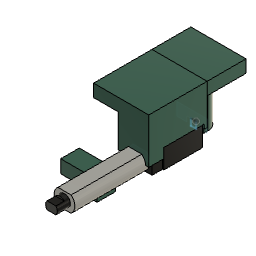
Actuator Casing (Autodesk Fusion 360 design; units mm, degrees)
Autodesk Fusion 360 part; units mm, degrees
note: some values were not read from the file. Chosen so that the rebuilt part matches the saved one: which bodies a step acts on; which pieces of a blend or face edit are solid. Set by a fixed rule: which sketch regions a step uses.
sketch "Sketch4" plane through (0, 0, 0) normal (0, 1, 0) x (1, 0, 0)
  line L0 (-5.3517, 0.0536) -> (-5.3517, 0) construction
  line L1 (-5.1362, -6.1335) -> (5.1362, -6.1335)
  line L2 (5.1029, 6.1612) -> (-5.1029, 6.1612)
  arc A0 (5.1362, -6.1335) -> (5.1029, 6.1612) centre (0, 0) ccw
  arc A1 (-5.1029, 6.1612) -> (-5.1362, -6.1335) centre (0, 0) ccw
  line L3 (-3.4975, -0.0044) -> (-3.4975, -3.0044) construction
  line L4 (-3.3853, -2.9647) -> (3.3222, -2.9647)
  line L5 (3.3222, 3.0353) -> (-3.3853, 3.0353)
  line L6 (-3.3853, 3.0353) -> (-3.3853, 2.9647)
  line L7 (-9.0073, 0.0216) -> (-9.0073, -7.4784) construction
  line L8 (0, 0) -> (-9.5, 0) construction
  line L9 (-9.5, 0) -> (-9.5, -7.4784) construction
  line L10 (-9.5, -7.4784) -> (9.5, -7.4784)
  line L11 (9.5, -7.4784) -> (9.5, 7.5216)
  line L12 (9.5, 7.5216) -> (-9.5, 7.5216)
  line L13 (-9.5, 7.5216) -> (-9.5, -7.4784)
  line L14 (-9.5, 7.5216) -> (-9.5, -7.4784)
  arc A2 (3.3853, -2.9647) -> (3.3222, 3.0353) centre (0, 0) ccw
  arc A3 (-3.3222, 3.0353) -> (-3.3853, -2.9647) centre (0, 0) ccw
  line L15 (3.3222, -2.9647) -> (3.3853, -2.9647)
  circle A4 centre (0, 0) radius 4.5
  line L16 (9.5, 7.5216) -> (10.5, 7.5216)
  line L17 (10.5, 7.5216) -> (10.5, -7.4784)
  line L18 (10.5, -7.4784) -> (9.5, -7.4784)
  line L19 (9.5, -7.4784) -> (9.5, 7.5216)
  dimension "d21" = 16
  dimension "d23" = 9
  dimension "d24" = 3
  dimension "d25" = 6
  dimension "d26" = 7.5
  dimension "d27" = 9.5
  dimension "d28" = 19
  dimension "d29" = 15
  dimension "d31" = 15
  dimension "d34" = 9
  dimension "d85" = 1
  dimension "d86" = 15
  constraint coincident A0.centre A1.centre
  constraint vertical L0
  constraint horizontal L1
  constraint horizontal L2
  constraint concentric A0 A1
  constraint vertical L3
  constraint horizontal L4
  constraint horizontal L5
  constraint vertical L6
  constraint vertical L7
  constraint perpendicular L7 L8
  constraint perpendicular L8 L9
  constraint horizontal L10
  constraint vertical L11
  constraint horizontal L12
  constraint vertical L13
  constraint vertical L14
  constraint coincident L4 A2.start
  constraint coincident L6.end A2
  constraint coincident L5 A3.start
  constraint concentric A2 A3
  constraint coincident L8 L0.end
  constraint concentric A1 A4
  constraint horizontal L16
  constraint vertical L17
  constraint horizontal L18
  constraint vertical L19
  measures "d21" diameter of A0
  measures "d23" diameter of A2
  measures "d24" distance of L3.start L3.end
  measures "d25" distance of L4.start L5.end
  measures "d26" distance of L7.start L7.end
  measures "d27" distance of A0.centre L8.end
  measures "d28" distance of L9.end L10.end
  measures "d29" distance of L9.end L12.end
  measures "d31" distance of L9.end L12.end
  measures "d34" diameter of A4
  measures "d85" distance of L11.end L16.end
  measures "d86" distance of L11.end L10.end
extrude "Extrude9" add sketch "Sketch4" against normal blind 68 contours L4 L5 A2 A3 L15 A4 makes body 1
extrude "Extrude10" add sketch "Sketch4" against normal blind 61.5 contours L4 L15 A4 | L5 A4 bodies 1
extrude "Extrude11" add sketch "Sketch4" against normal blind 58 contours L1 L2 A0 A1 bodies 1
extrude "Extrude12" add sketch "Sketch4" along normal blind 38 contours L10 L11 L12 L13 L14 L19 bodies 1
extrude "Extrude13" add sketch "Sketch4" along normal blind 30 from surface at 8 contours L1 L2 A0 A1 | L10 L11 L12 L13 L14 L19 | L11 L16 L17 L18 L19 bodies 1
sketch "Sketch5" plane through (0, 0, 0) normal (0, 0, 1) x (1, 0, 0)
  circle A0 centre (0, 43) radius 2.15
  line L0 (-5, 38) -> (-5, 43)
  line L1 (5, 38) -> (5, 43)
  arc A1 (5, 43) -> (-5, 43) centre (0, 43) ccw
  line L2 (-5, 38) -> (5, 38)
  dimension "d53" = 10
  dimension "d54" = 4.3
  constraint concentric A0 A1
  constraint tangent L0 A1
  constraint tangent L1 A1
  constraint horizontal L2
  measures "d53" diameter of A1
  measures "d54" diameter of A0
extrude "Extrude14" add sketch "Sketch5" along normal blind 4 and the other way blind 4 bodies 1
sketch "Sketch6" plane through (0, 38, 0) normal (0, 1, 0) x (-1, 0, 0)
  line L0 (9.5, 7.4784) -> (-10.5, 7.4784)
  line L1 (-10.5, -7.5216) -> (9.5, -7.5216)
  line L2 (9.5, 7.4784) -> (-10.5, 7.4784)
  line L3 (-10.5, 7.4784) -> (-10.5, -7.5216)
  line L4 (-10.5, -7.5216) -> (9.5, -7.5216)
  line L5 (9.5, -7.5216) -> (9.5, 7.4784)
  arc A0 (2.0616, 4) -> (-2.0616, 4) centre (0, 0) ccw
  line L6 (-5, 4) -> (-2.0616, 4)
  line L7 (2.0616, 4) -> (5, 4)
  line L8 (5, 4) -> (5, -4)
  line L9 (5, -4) -> (2.0616, -4)
  arc A1 (-2.0616, -4) -> (2.0616, -4) centre (0, 0) ccw
  line L10 (-2.0616, -4) -> (-5, -4)
  line L11 (-5, -4) -> (-5, 4)
  line L12 (-10.5, 7.4784) -> (-10.5, -7.5216)
  line L13 (9.5, -7.5216) -> (9.5, 7.4784)
  constraint horizontal L2
  constraint vertical L3
  constraint horizontal L4
  constraint vertical L5
  constraint coincident L1.start L3.end
  constraint coincident L0.start L2.start
sketch "Sketch7" plane through (0, 0, 2.9647) normal (0, 0, 1) x (-1, 0, 0)
  line L0 (-3.3853, 61.5) -> (3.3853, 61.5)
  line L1 (3.3853, 61.5) -> (3.3853, 68)
  line L2 (3.3853, 68) -> (-3.3853, 68)
  line L3 (-3.3853, 68) -> (-3.3853, 61.5)
copy_body "Body->Comp1" bodies 1 removing the originals makes body 2 in component "actuator"
sketch "Sketch5 (2)" plane through (0, 0, 0) normal (0, 0, 1) x (1, 0, 0) in component "casing 1"
  line L0 (13, 0) -> (-12, 0)
  line L1 (13, 38) -> (-12, 38)
  line L2 (-10, -58) -> (10.3853, -58)
  constraint horizontal L0
  constraint horizontal L1
  constraint horizontal L2
split "Split2" by plane through (0, 0, 0) normal (0, 1, 0) bodies 2 makes body 3 at (-3.1667, 15.3333, 7.4784) in component "actuator"
sketch "Sketch1" plane through (0, 0, 6.1335) normal (0, 0, 1) x (-1, 0, 0) in component "actuator"
  line L0 (-5.1362, 0) -> (5.1362, 0)
  line L1 (5.1362, 0) -> (5.1362, 58)
  line L2 (5.1362, 58) -> (-5.1362, 58)
  line L3 (-5.1362, 58) -> (-5.1362, 0)
  line L4 (-10.7245, 58) -> (12, 58)
  constraint horizontal L4
split "Split3" by curves path "Sketch1" along L4 bodies 2 makes body 4 at (-5.4286, -19.3333, 5.8763) in component "actuator"
sketch "Sketch2" plane through (0, 0, 7.4784) normal (0, 0, 1) x (-1, 0, 0) in component "actuator"
  line L0 (9.5, -38) -> (9.5, 0)
  line L1 (9.5, 0) -> (-9.5, 0)
  line L2 (-9.5, 0) -> (-9.5, -8)
  line L3 (-9.5, -8) -> (-10.5, -8)
  line L4 (-10.5, -8) -> (-10.5, -38)
  line L5 (-10.5, -38) -> (9.5, -38)
  line L6 (-12.8885, -38) -> (12, -38)
  constraint perpendicular L0 L6
split "Split4" by curves path "Sketch2" along L6 bodies 3 makes body 5 at (-4.9752, 43.4978, -1.3333) in component "actuator"
sketch "Sketch3" plane through (0, 0, 0) normal (0, 0, 1) x (1, 0, 0) in component "actuator"
sketch "Sketch12" plane through (0, 0, 0) normal (0, 0, 1) x (1, 0, 0) in component "casing 1"
  line L0 (10.5, 38) -> (4.5, 38)
  line L1 (8, 0) -> (9.5, 0)
  line L2 (-4.5, 38) -> (-9.5, 38)
  line L3 (-9.5, 38) -> (-9.5, 0)
  line L4 (-9.5, 0) -> (-8, 0)
  line L5 (-4.5, 38) -> (4.5, 38)
  line L6 (-8, 0) -> (8, 0)
  line L7 (10.5, 41.5) -> (4.5, 41.5)
  line L8 (-4.5, 41.5) -> (4.5, 41.5)
  line L9 (-4.5, 41.5) -> (-13, 41.5)
  line L10 (-13, 41.5) -> (-13, -3.5)
  line L11 (-13, -3.5) -> (-8, -3.5)
  line L12 (-8, -3.5) -> (8, -3.5)
  line L13 (8, -3.5) -> (9.5, -3.5)
  line L14 (10.5, 41.5) -> (10.5, -3.5)
  line L15 (10.5, -3.5) -> (9.5, -3.5)
  dimension "d117" = 3.5
  constraint coincident L2.start L5.start
  constraint coincident L0.end L5.end
  constraint coincident L4.end L6.start
  constraint coincident L1.start L6.end
  constraint perpendicular L13 L14
  constraint perpendicular L14 L15
extrude "Extrude10'" add sketch "Sketch12" along normal blind 10 separate body makes body 6 in component "casing 1"
combine "Combine3" operation cut target body 6 tool bodies 3 4 5 keep tools in component "casing 1"
sketch "Sketch13" plane through (0, 0, 0) normal (0, -1, 0) x (1, 0, 0) in component "casing 1"
  line L0 (-8, 0) -> (8, 0)
  arc A0 (8, 0) -> (5.1362, 6.1335) centre (0, 0) ccw
  line L1 (5.1362, 6.1335) -> (-5.1362, 6.1335)
  arc A1 (-5.1362, 6.1335) -> (-8, 0) centre (0, 0) ccw
sketch "Sketch14" plane through (0, 0, 3.0668) normal (0, -1, 0) x (1, 0, 0) in component "casing 1"
  line L0 (8.1565, -4.4312) -> (-8, -4.4312)
  line L1 (-8, -4.4312) -> (-8, 5)
  line L2 (-8, 5) -> (8.1565, 5)
  line L3 (8.1565, 5) -> (8.1565, -4.4312)
  constraint horizontal L0
  constraint vertical L1
  constraint horizontal L2
  constraint vertical L3
extrude "Extrude11'" cut sketch "Sketch14" against normal blind 38 bodies 6 in component "casing 1"
sketch "Sketch15" plane through (0, 41.5, 0) normal (0, 1, 0) x (-1, 0, 0) in component "casing 1"
  line L0 (5, 4) -> (5, 0)
  line L1 (5, 0) -> (13, 0)
  line L2 (13, 0) -> (13, 10)
  line L3 (13, 10) -> (-10.5, 10)
  line L4 (-10.5, 10) -> (-10.5, 0)
  line L5 (-10.5, 0) -> (-5, 0)
  line L6 (-5, 0) -> (-5, 4)
  line L7 (-5, 4) -> (-1.5403, 4)
  line L8 (-1.5403, 4) -> (-1.5403, 0)
  line L9 (-1.5403, 0) -> (1.5403, 0)
  line L10 (1.5403, 0) -> (1.5403, 4)
  line L11 (1.5403, 4) -> (5, 4)
  line L12 (2, -1) -> (-2, -1)
  line L13 (-2, -1) -> (-2, 4)
  line L14 (-2, 4) -> (2, 4)
  line L15 (2, 4) -> (2, -1)
  constraint horizontal L12
  constraint vertical L13
  constraint horizontal L14
  constraint vertical L15
  constraint coincident L7 L13.end
sketch "Sketch16" plane through (0, 0, 0) normal (0, 0, -1) x (1, 0, 0) in component "casing 1"
  arc A0 (1.5403, -41.5) -> (-1.5403, -41.5) centre (0, -43) ccw
  line L0 (-1.5403, -41.5) -> (1.5403, -41.5)
  line L1 (-1.8649, -40.1939) -> (2.2396, -40.1939)
  line L2 (2.2396, -40.1939) -> (2.2396, -42.4909)
  line L3 (2.2396, -42.4909) -> (-1.8649, -42.4909)
  line L4 (-1.8649, -42.4909) -> (-1.8649, -40.1939)
  constraint horizontal L1
  constraint vertical L2
  constraint horizontal L3
  constraint vertical L4
move_face "OffsetFaces1" offset -4 1 faces at (-0.4357, 41.431, 0) on bodies 6 in component "casing 1"
move_face "OffsetFaces2" offset -4.5 1 faces at (-5, 39.1667, 1.3333) on bodies 6 in component "casing 1"
move_face "OffsetFaces3" offset -5.5 1 faces at (5, 39.1667, 1.3333) on bodies 6 in component "casing 1"
sketch "Sketch17" plane through (0, 0, 10) normal (0, 0, 1) x (-1, 0, 0) in component "casing 1"
  line L0 (-10.5, -41.5) -> (13, -41.5)
  line L1 (13, -41.5) -> (13, 3.5)
  line L2 (13, 3.5) -> (-10.5, 3.5)
  line L3 (-10.5, 3.5) -> (-10.5, -41.5)
  line L4 (-10.5, 3.5) -> (-4.9498, 3.5)
  line L5 (-4.9498, 3.5) -> (-4.9498, -41.5)
  line L6 (-4.9498, -41.5) -> (-10.5, -41.5)
  line L7 (-10.5, -41.5) -> (-10.5, 3.5)
  constraint horizontal L4
  constraint vertical L5
  constraint horizontal L6
  constraint vertical L7
  constraint coincident L0 L5.end
  constraint coincident L2.end L3.start
extrude "Extrude13'" add sketch "Sketch17" along normal blind 20 contours L0 L2 L3 L4 L5 L6 L7 bodies 6 in component "casing 1"
sketch "Sketch18" plane through (4.9498, 0, 0) normal (-1, 0, 0) x (0, -1, 0) in component "casing 1"
  line L0 (-41.5, 10) -> (3.5, 10)
  line L1 (3.5, 10) -> (3.5, 30)
  line L2 (3.5, 30) -> (-41.5, 30)
  line L3 (-41.5, 30) -> (-41.5, 10)
  line L4 (3.5, 30) -> (-41.5, 30)
  line L5 (-41.5, 30) -> (-41.5, 25.3289)
  line L6 (-41.5, 25.3289) -> (3.5, 25.3289)
  line L7 (3.5, 25.3289) -> (3.5, 30)
  constraint horizontal L4
  constraint vertical L5
  constraint horizontal L6
  constraint vertical L7
  constraint coincident L3 L5.end
  constraint coincident L1.end L2.start
extrude "Extrude14'" add sketch "Sketch18" along normal blind 27 contours L1 L2 L3 L4 L5 L6 L7 bodies 6 in component "casing 1"
sketch "Sketch1 (2)" plane through (4.9498, 0, 0) normal (-1, 0, 0) x (0, -1, 0) in component "casing2"
  line L0 (3.5, 25.3289) -> (-41.5, 25.3289)
  line L1 (-41.5, 25.3289) -> (-41.5, 10)
  line L2 (-41.5, 10) -> (3.5, 10)
  line L3 (3.5, 10) -> (3.5, 25.3289)
  line L4 (23.5354, 14.7844) -> (31.8865, 14.7844)
  line L5 (31.8865, 14.7844) -> (31.8865, -18.9031)
  line L6 (31.8865, -18.9031) -> (23.5354, -18.9031)
  line L7 (23.5354, -18.9031) -> (23.5354, 14.7844)
  constraint horizontal L4
  constraint vertical L5
  constraint horizontal L6
  constraint vertical L7
extrude "Extrude1" add sketch "Sketch1 (2)" along normal blind 15 separate body contours L4 L5 L6 L7 makes body 7 in component "casing2"
combine "Combine1" operation cut target body 7 tool bodies 4 keep tools makes body 8 at (-3.4011, -31.8865, -14.6558) in component "casing2"
move_face "OffsetFaces1'" offset -10 1 faces at (-0.0502, -29.1028, -18.9031) on bodies 8 in component "casing2"
move_face "OffsetFaces2'" offset -8.6 1 faces at (-0.0502, -26.3191, 14.7844) on bodies 8 in component "casing2"
fillet "Fillet1" radius 9 1 edges at (-10.0502, -27.7109, -8.9031) on bodies 8 in component "casing2"
sketch "Sketch2 (2)" plane through (-10.0502, 0, 0) normal (-1, 0, 0) x (0, -1, 0) in component "casing2"
  line L0 (23.5354, 0.0969) -> (31.8865, 0.0969)
  line L1 (31.8865, 0.0969) -> (31.8865, 6.1844)
  line L2 (31.8865, 6.1844) -> (23.5354, 6.1844)
  line L3 (23.5354, 6.1844) -> (23.5354, 0.0969)
  line L4 (31.8865, 6.1844) -> (23.5354, 6.1844)
  line L5 (23.5354, 6.1844) -> (23.5354, 3.1406)
  line L6 (23.5354, 3.1406) -> (31.8865, 3.1406)
  line L7 (31.8865, 3.1406) -> (31.8865, 6.1844)
  constraint horizontal L4
  constraint vertical L5
  constraint horizontal L6
  constraint vertical L7
  constraint midpoint L3 L5.end
  constraint coincident L1.end L2.start
extrude "Extrude2" add sketch "Sketch2 (2)" along normal blind 13 contours L1 L2 L3 L4 L5 L6 L7 bodies 8 in component "casing2"
delete_face "DeleteFace1" 1 faces at (-1.7742, -26.3191, 6.1335) on bodies 8 in component "casing2"
move_face "OffsetFaces4" offset 15.5 1 faces at (-7.0167, 11.5, 10) on bodies 6 in component "casing 1"
move_face "OffsetFaces3'" offset 6 1 faces at (-12.725, -31.8865, 5.1698) on bodies 8 in component "casing2"
move_face "OffsetFaces4'" offset 7 1 faces at (-14.3835, -28.3191, 3.1406) on bodies 8 in component "casing2"
move_face "OffsetFaces5" offset 5 1 faces at (-0.3501, 11.5, 30) on bodies 6 in component "casing 1"
sketch "Sketch3 (2)" plane through (0, 41.5, 0) normal (0, 1, 0) x (-1, 0, 0) in component "casing2"
  line L0 (13, 25.3289) -> (22.0502, 25.3289)
  line L1 (22.0502, 25.3289) -> (22.0502, 35)
  line L2 (22.0502, 35) -> (-10.5, 35)
  line L3 (-10.5, 35) -> (-10.5, 4)
  line L4 (-10.5, 4) -> (9.5, 4)
  line L5 (9.5, 4) -> (9.5, 0)
  line L6 (9.5, 0) -> (13, 0)
  line L7 (13, 0) -> (13, 25.3289)
  line L8 (22.0502, 35) -> (-10.5, 35)
  line L9 (-10.5, 35) -> (-10.5, 25.3289)
  line L10 (-10.5, 25.3289) -> (22.0502, 25.3289)
  line L11 (22.0502, 25.3289) -> (22.0502, 35)
  constraint horizontal L8
  constraint vertical L9
  constraint horizontal L10
  constraint vertical L11
  constraint coincident L3 L9.end
  constraint coincident L1.end L2.start
extrude "Extrude3" add sketch "Sketch3 (2)" along normal blind 20 separate body contours L0 L1 L2 L3 L8 L9 L10 L11 makes body 9 in component "casing2"
move_face "OffsetFaces6" offset -1.3 1 faces at (1.7188, 38, 6.7112) on bodies 6 in component "casing 1"
sketch "Sketch4 (2)" plane through (0, 0, 0) normal (0, 0, -1) x (1, 0, 0) in component "casing2"
  line L0 (-9.5, -38) -> (-9.5, 0)
  line L1 (-9.5, 0) -> (-8, 0)
  line L2 (-8, 0) -> (-8, 3.5)
  line L3 (-8, 3.5) -> (-13, 3.5)
  line L4 (-13, 3.5) -> (-13, -41.5)
  line L5 (-13, -41.5) -> (-9.5, -41.5)
  line L6 (-9.5, -41.5) -> (-9.5, -38)
  line L7 (-9.5, -41.5) -> (-13, -41.5)
  line L8 (-13, -41.5) -> (-13, -34.0091)
  line L9 (-13, -34.0091) -> (-9.5, -34.0091)
  line L10 (-9.5, -34.0091) -> (-9.5, -41.5)
  constraint horizontal L7
  constraint vertical L8
  constraint horizontal L9
  constraint vertical L10
  constraint coincident L4 L8.end
  constraint coincident L5.end L6.start
extrude "Extrude4" add sketch "Sketch4 (2)" along normal blind 7.5 separate body contours L0 L4 L5 L6 L7 L8 L9 L10 makes body 10 in component "casing2"
sketch "Sketch5 (3)" plane through (-9.5, 0, 0) normal (1, 0, 0) x (0, 1, 0) in component "casing2"
  line L0 (41.5, 0) -> (34.0091, 0)
  line L1 (34.0091, 0) -> (34.0091, -7.5)
  line L2 (34.0091, -7.5) -> (41.5, -7.5)
  line L3 (41.5, -7.5) -> (41.5, 0)
  line L4 (41.5, -7.5) -> (39.6483, -7.5)
  line L5 (39.6483, -7.5) -> (39.6483, -4.4617)
  line L6 (39.6483, -4.4617) -> (41.5, -4.4617)
  line L7 (41.5, -4.4617) -> (41.5, -7.5)
  constraint horizontal L4
  constraint vertical L5
  constraint horizontal L6
  constraint vertical L7
  constraint coincident L2.end L3.start
extrude "Extrude5" add sketch "Sketch5 (3)" along normal blind 13 contours L2 L3 L4 L5 L6 L7 bodies 10 in component "casing2"
copy_body "CutPasteBodies1" bodies 9 removing the originals makes body 11 in component "casing 1"
move_face "OffsetFaces7" offset 10 2 faces at (-22.0502, 48.1667, 28.5526) (-22.0502, 11.5, 28.5526) on bodies 6 11 in component "casing 1"
sketch "Sketch19" plane through (0, 0, 4) normal (0, 0, -1) x (1, 0, 0) in component "casing 1"
  line L0 (-9.5, -39.3) -> (-9.5, -41.5)
  line L1 (-9.5, -41.5) -> (10.5, -41.5)
  line L2 (10.5, -41.5) -> (10.5, -39.3)
  line L3 (10.5, -39.3) -> (-9.5, -39.3)
  line L4 (-5, -38) -> (-5, -43)
  arc A0 (-5, -43) -> (5, -43) centre (0, -43) ccw
  line L5 (5, -43) -> (5, -38)
  line L6 (-5.6727, -38) -> (-5.6727, -43)
  arc A1 (-5.6727, -43) -> (5.6727, -43) centre (0, -43) ccw
  line L7 (5.6727, -43) -> (5.6727, -38)
  line L8 (-9.4287, -38) -> (-9.4287, -43)
  arc A2 (-9.4287, -43) -> (9.4287, -43) centre (0, -43) ccw
  line L9 (9.4287, -43) -> (9.4287, -38)
  line L10 (-9.4287, -38) -> (-5.6727, -38)
  line L11 (5.6727, -38) -> (9.4287, -38)
  dimension "d151" = 0.6727
  dimension "d152" = 4.4287
  constraint perpendicular L6 L10
  constraint perpendicular L9 L11
extrude "Extrude15" add sketch "Sketch19" along normal blind 3.5 contours L3 L6 L8 L10 | L1 L3 L6 L8 | L1 L6 A1 L7 L8 A2 L9 | L1 L3 L7 L9 | L3 L7 L9 L11 bodies 6 in component "casing 1"
move_face "OffsetFaces8" offset 23 1 faces at (-8.1767, 42, 4) on bodies 6 in component "casing 1"
move_face "OffsetFaces9" offset 10 1 faces at (-3.6834, 61.5, 28.5526) on bodies 11 in component "casing 1"
move_face "OffsetFaces10" offset -2 1 faces at (-8.1767, 38, 2.8333) on bodies 6 in component "casing 1"
move_face "OffsetFaces11" offset -2 1 faces at (6.9247, 38, 2.8333) on bodies 6 in component "casing 1"
component "casing 1" placed x (1, 0, 0) y (0, 1, 0) z (0, 0, 1) at (0, 0, 0)
component "actuator" placed x (1, 0, 0) y (0, 1, 0) z (0, 0, 1) at (0, 0, 0)
component "casing2" placed x (1, 0, 0) y (0, 1, 0) z (0, 0, 1) at (0, 0, 0)
hidden bodies 7
